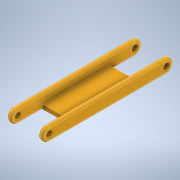
# Autodesk Inventor part: Thick Leg
Saved by Autodesk Inventor 2022.4 (Build 264492000, 492)
## iProperties
Created: 2024-04-25
Part Number: Thick Leg
Material: Generic
Document SubType Name: Modeling
Designer: t60147996
Density: 1 g/cm^3
Appearance: Weld - Brass
Author: t60147996
Autodesk Inventor part; units mm, degrees
ref_plane "YZ Plane" through (0, 0, 0) normal (1, 0, 0) x (0, 1, 0)
ref_plane "XZ Plane" through (0, 0, 0) normal (0, 1, 0) x (-1, 0, 0)
ref_plane "XY Plane" through (0, 0, 0) normal (0, 0, 1) x (1, 0, 0)
sketch "Sketch1" plane through (0, 0, 0) normal (0, 1, 0) x (-1, 0, 0)
  line L0 (25.4, 47.498) -> (-25.4, 47.498)
  line L1 (-25.4, 47.498) -> (-25.4, -47.498)
  line L2 (-25.4, -47.498) -> (25.4, -47.498)
  line L3 (25.4, -47.498) -> (25.4, 47.498)
  line L4 (25.4, 47.498) -> (-25.4, -47.498) construction
  line L5 (-25.4, 47.498) -> (25.4, -47.498) construction
  point P0 (0, 0)
  dimension "d0" = 50.8
  dimension "d1" = 94.996
  constraints: 12 end point, 2 midpoint, 2 parallel, 1 horizontal, 1 perpendicular
  measures "d0" distance of L2.end L1.end
  measures "d1" distance of L1.end L0.end
extrude "Extrusion1" add sketch "Sketch1" along normal blind 6.35
sketch "Sketch2" plane through (25.4, 0, 47.498) normal (1, 0, 0) x (0, 0, -1)
  line L0 (-35.052, 19.05) -> (130.048, 19.05)
  line L1 (130.048, 19.05) -> (130.048, 0)
  line L2 (130.048, 0) -> (-35.052, 0)
  line L3 (-35.052, 0) -> (-35.052, 19.05)
  line L4 (-35.052, 19.05) -> (130.048, 0) construction
  line L5 (130.048, 19.05) -> (-35.052, 0) construction
  line L6 (0, 0) -> (94.996, 0) projected
  circle A0 centre (-35.052, 9.525) radius 9.525
  circle A1 centre (130.048, 9.525) radius 9.525
  point P0 (47.498, 0)
  point P1 (47.498, 9.525)
  point P2 (47.498, 0)
  dimension "d4" = 165.1
  dimension "d5" = 19.05
  constraints: 12 end point, 6 midpoint, 2 parallel, 1 horizontal, 1 perpendicular, 6 other
  measures "d4" distance of L1.end L2.end
  measures "d5" distance of L0.end L1.end
extrude "Extrusion2" add sketch "Sketch2" against normal blind 6.35
fillet "Fillet1" radius 2.54 9 edges at (19.05, 0, -65.024) (19.05, 19.05, 0) (19.05, 9.525, 92.075) (19.05, 0, 65.024) (19.05, 9.525, -92.075) (25.4, 19.05, 0) (25.4, 9.525, 92.075) (25.4, 0, 0) (25.4, 9.525, -92.075)
mirror "Mirror1" about plane through (0, 0, 0) normal (1, 0, 0) of "Extrusion2", "Fillet1"
sketch "Sketch3" plane through (25.4, 9.525, 82.55) normal (1, 0, 0) x (0, 0, -1)
  arc A0 (165.1, -6.985) -> (165.1, 6.985) centre (165.1, 0) ccw projected
  point P0 (82.55, -9.525)
  point P1 (0, 0)
  constraints: 1 coincident
hole "Hole1" at (25.4, 9.525, 82.55) at (25.4, 9.525, -82.55) direction (-1, 0, 0) diameter 8.89 end through all
body "Solid1"
